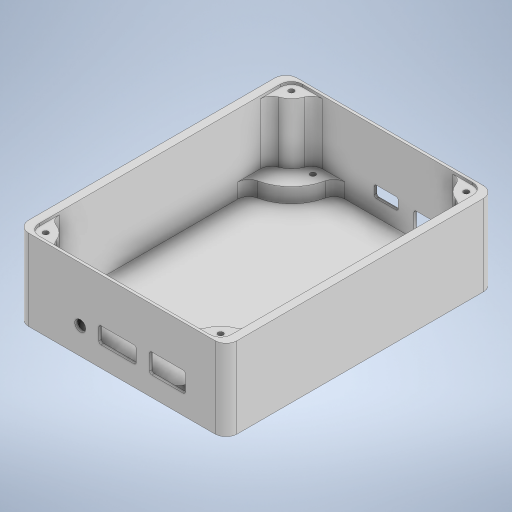
# Autodesk Inventor part: PrismGCNew
Saved by Autodesk Inventor 2024 (Build 280153000, 153)
## iProperties
Created: 2023-08-08
Part Number: PrismGCNew
Material: 常规
Document SubType Name: Modeling
Designer: liyuxuan
Density: 1 g/cm^3
Appearance: 默认
Author: liyuxuan
Autodesk Inventor part; units mm, degrees
ref_plane "YZ Plane" through (0, 0, 0) normal (1, 0, 0) x (0, 1, 0)
ref_plane "XZ Plane" through (0, 0, 0) normal (0, 1, 0) x (-1, 0, 0)
ref_plane "XY Plane" through (0, 0, 0) normal (0, 0, 1) x (1, 0, 0)
sketch "草图1" plane through (0, 0, 0) normal (0, 1, 0) x (-1, 0, 0)
  line L0 (-47.7, 61.39) -> (47.7, 61.39)
  line L1 (47.7, 61.39) -> (47.7, -61.39)
  line L2 (47.7, -61.39) -> (-47.7, -61.39)
  line L3 (-47.7, -61.39) -> (-47.7, 61.39)
  line L4 (-47.7, 61.39) -> (47.7, -61.39) construction
  line L5 (47.7, 61.39) -> (-47.7, -61.39) construction
  line L6 (-44, 60.19) -> (44, 60.19)
  line L7 (44, 60.19) -> (44, -60.19)
  line L8 (44, -60.19) -> (-44, -60.19)
  line L9 (-44, -60.19) -> (-44, 60.19)
  line L10 (-44, 60.19) -> (44, -60.19) construction
  line L11 (44, 60.19) -> (-44, -60.19) construction
  arc A0 (24, 60.19) -> (44, 40.19) centre (44, 60.19) ccw
  line L12 (44, 60.19) -> (24, 60.19) construction
  line L13 (44, 60.19) -> (44, 40.19) construction
  arc A1 (34, 60.19) -> (44, 50.19) centre (44, 60.19) ccw
  line L14 (44, 60.19) -> (34, 60.19) construction
  line L15 (44, 60.19) -> (44, 50.19) construction
  line L16 (44, 0) -> (-44, 0)
  line L17 (0, 60.19) -> (0, -60.19)
  circle A2 centre (40, 56.19) radius 1.25
  circle A3 centre (29.848, 55.88) radius 1.25
  arc A4 (44, -40.19) -> (24, -60.19) centre (44, -60.19) ccw
  arc A5 (44, -50.19) -> (34, -60.19) centre (44, -60.19) ccw
  circle A6 centre (40, -56.19) radius 1.25
  circle A7 centre (29.848, -55.88) radius 1.25
  arc A8 (-44, 40.19) -> (-24, 60.19) centre (-44, 60.19) ccw
  arc A9 (-44, 50.19) -> (-34, 60.19) centre (-44, 60.19) ccw
  circle A10 centre (-40, 56.19) radius 1.25
  circle A11 centre (-29.848, 55.88) radius 1.25
  arc A12 (-24, -60.19) -> (-44, -40.19) centre (-44, -60.19) ccw
  circle A13 centre (-29.848, -55.88) radius 1.25
  arc A14 (-34, -60.19) -> (-44, -50.19) centre (-44, -60.19) ccw
  circle A15 centre (-40, -56.19) radius 1.25
  point P0 (0, 0)
  point P1 (-44, -50.19)
  point P2 (-34, -60.19)
  point P3 (-24, -60.19)
  point P4 (-44, -40.19)
  point P5 (-34, 60.19)
  point P6 (-44, 50.19)
  point P7 (-44, 40.19)
  point P8 (-24, 60.19)
  point P9 (44, -50.19)
  dimension "d0" = 122.78
  dimension "d1" = 95.4
  dimension "d2" = 120.38
  dimension "d3" = 88
  dimension "d4" = 20
  dimension "d5" = 90
  dimension "d6" = 10
  dimension "d7" = 90
  dimension "d8" = 55.88
  dimension "d9" = 29.848
  dimension "d10" = 4
  dimension "d11" = 4
  dimension "d12" = 2.5
  dimension "d13" = 2.5
  constraints: 36 end point, 30 symmetric about line, 16 centre point, 16 point on circle, 13 coincident, 9 midpoint, 4 parallel, 2 horizontal, 2 perpendicular, 1 point on line, 12 other
  measures "d0" distance of L0.end L1.end
  measures "d1" distance of L0.start L0.end
  measures "d2" distance of L6.end L7.end
  measures "d3" distance of L6.start L6.end
  measures "d4" radius of A0
  measures "d5" angle of L12 L13
  measures "d6" radius of A1
  measures "d7" angle of L14 L15
  measures "d8" vertical distance of point (0, 0) point (29.848, 55.88)
  measures "d9" horizontal distance of point (29.848, 55.88) point (0, 0)
  measures "d10" distance from line of L12 point (40, 56.19)
  measures "d11" distance from line of L7 point (40, 56.19)
  measures "d12" diameter of A2
  measures "d13" diameter of A3
extrude "拉伸1" add sketch "草图1" along normal blind 37 contours L0 L1 L2 L3
extrude "拉伸2" add sketch "草图1" along normal blind 1.2 contours L6 A9 L9 | L6 A8 L9 A9 | L6 L17 L16 L9 A8 | L6 A0 L7 L16 L17 | L16 L17 L8 A12 L9 | L6 A1 L7 A0 | L16 L7 A4 L8 L17 | A12 L8 A14 L9 | L6 L7 A1 | A14 L8 L9 | L7 A5 L8 A4 | L7 L8 A5 | A2 | A3 | A6 | A7 | A10 | A11 | A13 | A15
extrude "拉伸3" add sketch "草图1" along normal blind 8 contours L6 A8 L9 A9 | L6 A1 L7 A0 | A12 L8 A14 L9 | L7 A5 L8 A4 | A3 | A7 | A11 | A13
extrude "拉伸4" add sketch "草图1" along normal blind 35.8 contours L6 A9 L9 | L6 L7 A1 | A14 L8 L9 | L7 L8 A5 | A2 | A6 | A10 | A15
sketch "草图3" plane through (0, 8, 0) normal (0, 1, 0) x (1, 0, 0)
  arc A0 (44, -50.19) -> (34, -60.19) centre (44, -60.19) ccw projected
  line L0 (44, -40.19) -> (44, -50.19) projected
  arc A1 (44, -40.19) -> (24, -60.19) centre (44, -60.19) ccw projected
  line L1 (-24, -60.19) -> (24, -60.19) projected
  arc A2 (-24, -60.19) -> (-44, -40.19) centre (-44, -60.19) ccw projected
  line L2 (-44, 40.19) -> (-44, -40.19) projected
  arc A3 (-44, 40.19) -> (-24, 60.19) centre (-44, 60.19) ccw projected
  line L3 (24, 60.19) -> (-24, 60.19) projected
  line L4 (34, 60.19) -> (24, 60.19) projected
  arc A4 (34, 60.19) -> (44, 50.19) centre (44, 60.19) ccw projected
  line L5 (44, 50.19) -> (44, 40.19) projected
  arc A5 (24, 60.19) -> (44, 40.19) centre (44, 60.19) ccw projected
  line L6 (24, -60.19) -> (34, -60.19) projected
  line L7 (44, -40.19) -> (44, 40.19) projected
  line L8 (-34, -60.19) -> (-24, -60.19) projected
  arc A6 (-34, -60.19) -> (-44, -50.19) centre (-44, -60.19) ccw projected
  line L9 (-44, -50.19) -> (-44, -40.19) projected
  line L10 (-44, 40.19) -> (-44, 50.19) projected
  arc A7 (-44, 50.19) -> (-34, 60.19) centre (-44, 60.19) ccw projected
  line L11 (-24, 60.19) -> (-34, 60.19) projected
  line L12 (47.7, 61.39) -> (47.7, -61.39) projected
  line L13 (47.7, -61.39) -> (-47.7, -61.39) projected
  line L14 (-47.7, -61.39) -> (-47.7, 61.39) projected
  line L15 (-47.7, 61.39) -> (47.7, 61.39) projected
  line L16 (-44, 0) -> (44, 0) projected
  line L17 (0, -60.19) -> (0, 60.19) projected
  arc A8 (-24, -60.19) -> (-44, -40.19) centre (-44, -60.19) ccw projected
  arc A9 (44, -50.19) -> (34, -60.19) centre (44, -60.19) ccw projected
  line L18 (44, -40.19) -> (44, -50.19) projected
  arc A10 (44, -40.19) -> (24, -60.19) centre (44, -60.19) ccw projected
  line L19 (-24, -60.19) -> (24, -60.19) projected
  arc A11 (-24, -60.19) -> (-44, -40.19) centre (-44, -60.19) ccw projected
  line L20 (-44, 40.19) -> (-44, -40.19) projected
  arc A12 (-44, 40.19) -> (-24, 60.19) centre (-44, 60.19) ccw projected
  line L21 (24, 60.19) -> (-24, 60.19) projected
  line L22 (34, 60.19) -> (24, 60.19) projected
  arc A13 (34, 60.19) -> (44, 50.19) centre (44, 60.19) ccw projected
  line L23 (44, 50.19) -> (44, 40.19) projected
  arc A14 (24, 60.19) -> (44, 40.19) centre (44, 60.19) ccw projected
  line L24 (24, -60.19) -> (34, -60.19) projected
  line L25 (44, -40.19) -> (44, 40.19) projected
  line L26 (-34, -60.19) -> (-24, -60.19) projected
  arc A15 (-34, -60.19) -> (-44, -50.19) centre (-44, -60.19) ccw projected
  line L27 (-44, -50.19) -> (-44, -40.19) projected
  line L28 (-44, 40.19) -> (-44, 50.19) projected
  arc A16 (-44, 50.19) -> (-34, 60.19) centre (-44, 60.19) ccw projected
  line L29 (-24, 60.19) -> (-34, 60.19) projected
  line L30 (47.7, 61.39) -> (47.7, -61.39) projected
  line L31 (47.7, -61.39) -> (-47.7, -61.39) projected
  line L32 (-47.7, -61.39) -> (-47.7, 61.39) projected
  line L33 (-47.7, 61.39) -> (47.7, 61.39) projected
  point P0 (0, 0)
  point P1 (-29.848, -55.88)
  point P2 (-29.848, -55.88)
  point P3 (-29.848, 55.88)
  point P4 (29.848, -55.88)
  point P5 (29.848, 55.88)
  constraints: 3 symmetric about line, 1 coincident
hole "孔3" at (-29.848, 8, 55.88) at (-29.848, 8, -55.88) at (29.848, 8, 55.88) at (29.848, 8, -55.88) direction (0, -1, 0) diameter 2.459 depth 6 tip angle 118 thread size "M3x0.5" designation "M3" class "6H" standard "GB Metric profile"
sketch "草图6" plane through (0, 35.8, 0) normal (0, 1, 0) x (1, 0, 0)
  arc A0 (44, -40.19) -> (24, -60.19) centre (44, -60.19) ccw projected
  line L0 (44, 40.19) -> (44, -40.19) projected
  arc A1 (24, 60.19) -> (44, 40.19) centre (44, 60.19) ccw projected
  line L1 (-24, 60.19) -> (24, 60.19) projected
  arc A2 (-44, 40.19) -> (-24, 60.19) centre (-44, 60.19) ccw projected
  line L2 (-44, -40.19) -> (-44, 40.19) projected
  arc A3 (-24, -60.19) -> (-44, -40.19) centre (-44, -60.19) ccw projected
  line L3 (24, -60.19) -> (-24, -60.19) projected
  arc A4 (44, -50.19) -> (34, -60.19) centre (44, -60.19) ccw projected
  line L4 (44, -50.19) -> (44, -60.19) projected
  line L5 (44, -60.19) -> (34, -60.19) projected
  line L6 (-34, -60.19) -> (34, -60.19) projected
  arc A5 (-34, -60.19) -> (-44, -50.19) centre (-44, -60.19) ccw projected
  line L7 (-44, 50.19) -> (-44, -50.19) projected
  arc A6 (-44, 50.19) -> (-34, 60.19) centre (-44, 60.19) ccw projected
  line L8 (34, 60.19) -> (-34, 60.19) projected
  arc A7 (34, 60.19) -> (44, 50.19) centre (44, 60.19) ccw projected
  line L9 (44, -50.19) -> (44, 50.19) projected
  line L10 (-34, -60.19) -> (-44, -60.19) projected
  line L11 (-44, -60.19) -> (-44, -50.19) projected
  line L12 (-44, 50.19) -> (-44, 60.19) projected
  line L13 (-44, 60.19) -> (-34, 60.19) projected
  line L14 (34, 60.19) -> (44, 60.19) projected
  line L15 (44, 60.19) -> (44, 50.19) projected
  line L16 (47.7, 61.39) -> (47.7, -61.39) projected
  line L17 (47.7, -61.39) -> (-47.7, -61.39) projected
  line L18 (-47.7, -61.39) -> (-47.7, 61.39) projected
  line L19 (-47.7, 61.39) -> (47.7, 61.39) projected
  arc A8 (44, -50.19) -> (34, -60.19) centre (44, -60.19) ccw projected
  line L20 (44, -50.19) -> (44, -60.19) projected
  line L21 (44, -60.19) -> (34, -60.19) projected
  line L22 (-34, -60.19) -> (34, -60.19) projected
  arc A9 (-34, -60.19) -> (-44, -50.19) centre (-44, -60.19) ccw projected
  line L23 (-44, 50.19) -> (-44, -50.19) projected
  arc A10 (-44, 50.19) -> (-34, 60.19) centre (-44, 60.19) ccw projected
  line L24 (34, 60.19) -> (-34, 60.19) projected
  arc A11 (34, 60.19) -> (44, 50.19) centre (44, 60.19) ccw projected
  line L25 (44, -50.19) -> (44, 50.19) projected
  line L26 (-34, -60.19) -> (-44, -60.19) projected
  line L27 (-44, -60.19) -> (-44, -50.19) projected
  line L28 (-44, 50.19) -> (-44, 60.19) projected
  line L29 (-44, 60.19) -> (-34, 60.19) projected
  line L30 (34, 60.19) -> (44, 60.19) projected
  line L31 (44, 60.19) -> (44, 50.19) projected
  line L32 (-44, 0) -> (44, 0) projected
  line L33 (0, -60.19) -> (0, 60.19) projected
  line L34 (47.7, 61.39) -> (47.7, -61.39) projected
  line L35 (47.7, -61.39) -> (-47.7, -61.39) projected
  line L36 (-47.7, -61.39) -> (-47.7, 61.39) projected
  line L37 (-47.7, 61.39) -> (47.7, 61.39) projected
  point P0 (0, 0)
  point P1 (-40, -56.19)
  point P2 (-40, 56.19)
  point P3 (40, -56.19)
  point P4 (40, 56.19)
  dimension "d50" = 4
  dimension "d51" = 4
  constraints: 3 symmetric about line
  measures "d50" distance from line of L10 point (-40, -56.19)
  measures "d51" distance from line of L11 point (-40, -56.19)
hole "孔5" at (-40, 35.8, 56.19) at (-40, 35.8, -56.19) at (40, 35.8, 56.19) at (40, 35.8, -56.19) direction (0, -1, 0) diameter 2.459 depth 6 tip angle 118 thread size "M3x0.5" designation "M3" class "6H" standard "GB Metric profile"
fillet "面圆角1" radius 5 1 edges at (44, 36.4, 60.19)
fillet "面圆角2" radius 5 1 edges at (47.7, 18.5, 61.39)
fillet "面圆角3" radius 5 1 edges at (-44, 36.4, -60.19)
fillet "面圆角4" radius 5 1 edges at (44, 36.4, -60.19)
fillet "面圆角5" radius 5 1 edges at (-44, 36.4, 60.19)
fillet "面圆角6" radius 5 1 edges at (47.7, 18.5, -61.39)
fillet "面圆角7" radius 5 1 edges at (-47.7, 18.5, 61.39)
fillet "面圆角8" radius 5 1 edges at (-47.7, 18.5, -61.39)
fillet "面圆角9" radius 5 1 edges at (-44, 21.9, -50.19)
fillet "面圆角10" radius 5 1 edges at (-34, 21.9, -60.19)
fillet "面圆角11" radius 5 1 edges at (-44, 4.6, -40.19)
fillet "面圆角12" radius 5 1 edges at (-24, 4.6, -60.19)
fillet "面圆角13" radius 5 1 edges at (24, 4.6, -60.19)
fillet "面圆角14" radius 5 1 edges at (44, 4.6, -40.19)
fillet "面圆角15" radius 5 1 edges at (34, 21.9, -60.19)
fillet "面圆角16" radius 5 1 edges at (44, 21.9, -50.19)
fillet "面圆角17" radius 5 1 edges at (44, 21.9, 50.19)
fillet "面圆角18" radius 5 1 edges at (34, 21.9, 60.19)
fillet "面圆角19" radius 5 1 edges at (44, 4.6, 40.19)
fillet "面圆角20" radius 5 1 edges at (24, 4.6, 60.19)
fillet "面圆角21" radius 5 1 edges at (-24, 4.6, 60.19)
fillet "面圆角22" radius 5 1 edges at (-44, 4.6, 40.19)
fillet "面圆角23" radius 5 1 edges at (-34, 21.9, 60.19)
fillet "面圆角24" radius 5 1 edges at (-44, 21.9, 50.19)
sketch "草图7" plane through (42.7, 0, 61.39) normal (0, 0, 1) x (1, 0, 0)
  line L0 (-83.3667, 8) -> (-83.3667, 8) projected
  line L1 (-83.3667, 8) -> (-77.2719, 8) projected
  line L2 (-77.2719, 8) -> (-72.5579, 8) projected
  line L3 (-62.2051, 8) -> (-72.5579, 8) projected
  line L4 (-62.2051, 8) -> (-67.1041, 8) projected
  line L5 (-67.1041, 8) -> (-86.7, 8) projected
  line L6 (-86.7, 8) -> (-86.7, 8) projected
  line L7 (-73.7775, 8) -> (-71.3185, 8) projected
  line L8 (-12.8421, 8) -> (-8.1281, 8) projected
  line L9 (-8.1281, 8) -> (-2.0333, 8) projected
  line L10 (-2.0333, 8) -> (1.3, 8) projected
  line L11 (1.3, 8) -> (-2.7, 8) projected
  line L12 (-2.7, 8) -> (-18.2959, 8) projected
  line L13 (-23.1949, 8) -> (-18.2959, 8) projected
  line L14 (-12.8421, 8) -> (-23.1949, 8) projected
  line L15 (-14.0815, 8) -> (-11.6225, 8) projected
  line L16 (-14.0815, 8) -> (-11.6225, 8) projected
  line L17 (-73.7775, 8) -> (-71.3185, 8) projected
  line L18 (-86.7, 1.2) -> (-82.7, 1.2) projected
  line L19 (-82.7, 1.2) -> (-67.1041, 1.2) projected
  line L20 (-67.1041, 1.2) -> (-62.2051, 1.2) projected
  line L21 (-23.1949, 1.2) -> (-62.2051, 1.2) projected
  line L22 (-23.1949, 1.2) -> (-18.2959, 1.2) projected
  line L23 (-18.2959, 1.2) -> (-2.7, 1.2) projected
  line L24 (-2.7, 1.2) -> (1.3, 1.2) projected
  line L25 (1.3, 1.2) -> (-2.7, 1.2) projected
  line L26 (-2.7, 1.2) -> (-18.2959, 1.2) projected
  line L27 (-18.2959, 1.2) -> (-23.1949, 1.2) projected
  line L28 (-62.2051, 1.2) -> (-23.1949, 1.2) projected
  line L29 (-62.2051, 1.2) -> (-67.1041, 1.2) projected
  line L30 (-67.1041, 1.2) -> (-82.7, 1.2) projected
  line L31 (-82.7, 1.2) -> (-86.7, 1.2) projected
  line L32 (-90.4, 37) -> (-85.4, 37) projected
  line L33 (0, 37) -> (0, 0) projected
  line L34 (-85.4, 37) -> (0, 0)
  line L35 (-85.4, 0) -> (-85.4, 37) projected
  line L36 (0, 37) -> (-84.5262, -1.8989)
  line L37 (-85.4, 9.6) -> (0, 9.6)
  line L38 (-40.2, 18.5) -> (-42.7, 9.6)
  line L39 (-86.7, 8) -> (-83.3667, 8) projected
  line L40 (-86.7, 8) -> (-2.7, 8)
  line L41 (-13.585, 18.05) -> (-29.985, 18.05)
  line L42 (-29.985, 18.05) -> (-29.985, 8.95)
  line L43 (-29.985, 8.95) -> (-13.585, 8.95)
  line L44 (-13.585, 8.95) -> (-13.585, 18.05)
  line L45 (-13.585, 18.05) -> (-29.985, 8.95) construction
  line L46 (-29.985, 18.05) -> (-13.585, 8.95) construction
  line L47 (-44.645, 16.85) -> (-44.645, 9.3)
  line L48 (-36.095, 16.85) -> (-53.195, 16.85)
  line L49 (-53.195, 16.85) -> (-53.195, 9.3)
  line L50 (-53.195, 9.3) -> (-36.095, 9.3)
  line L51 (-36.095, 9.3) -> (-36.095, 16.85)
  line L52 (-36.095, 16.85) -> (-53.195, 9.3) construction
  line L53 (-53.195, 16.85) -> (-36.095, 9.3) construction
  circle A0 centre (-61.663, 12.1) radius 2.5
  point P0 (-42.7, 0)
  point P1 (-24.285, 9.6)
  point P2 (-21.785, 8)
  point P3 (-21.785, 8.95)
  point P4 (-21.785, 18.05)
  point P5 (-21.785, 13.5)
  point P6 (-47.145, 9.6)
  point P7 (-44.645, 8)
  point P8 (-44.645, 13.075)
  point P9 (-64.163, 9.6)
  point P10 (-61.663, 8)
  dimension "d84" = 1.6
  dimension "d85" = 18.415
  dimension "d86" = 0.95
  dimension "d87" = 10.05
  dimension "d88" = 16.4
  dimension "d89" = 4.445
  dimension "d90" = 1.3
  dimension "d91" = 8.85
  dimension "d92" = 17.1
  dimension "d93" = 21.463
  dimension "d94" = 4.1
  dimension "d95" = 5
  constraints: 34 end point, 8 point on line, 6 midpoint, 4 parallel, 3 perpendicular, 2 coincident, 2 horizontal, 1 centre point, 1 collinear, 1 vertical, 5 other
  measures "d84" distance between parallel lines of L37 L3
  measures "d85" distance of point (-24.285, 9.6) L38.end
  measures "d86" distance of point (-21.785, 8.95) point (-21.785, 8)
  measures "d87" distance of point (-21.785, 8) point (-21.785, 18.05)
  measures "d88" distance of L43.end L42.end
  measures "d89" distance of point (-47.145, 9.6) point (-42.7, 9.6)
  measures "d90" distance of L47.end point (-44.645, 8)
  measures "d91" distance of point (-44.645, 8) L47.start
  measures "d92" distance of L50.end L49.end
  measures "d93" distance of point (-64.163, 9.6) L38.end
  measures "d94" distance of point (-61.663, 8) point (-61.663, 12.1)
  measures "d95" diameter of A0
extrude "拉伸5" cut sketch "草图7" against normal blind 20 contours A0 | L48 L38 L37 L47 L36 | L36 L47 L48 | L49 L48 L47 L36 | L36 L47 L37 L49 | L37 L47 L50 L49 | L48 L51 L34 | L34 L51 L37 L38 L48 | L37 L51 L50 L47 | L42 L41 L44 L37 L34 | L34 L37 L42 | L44 L43 L34 L37 | L43 L42 L37 L34
fillet "面圆角25" radius 1 1 edges at (-10.495, 16.85, 60.79)
fillet "面圆角26" radius 1 1 edges at (6.605, 16.85, 60.79)
fillet "面圆角27" radius 1 1 edges at (6.605, 9.3, 60.79)
fillet "面圆角28" radius 1 1 edges at (-10.495, 9.3, 60.79)
fillet "面圆角29" radius 1 1 edges at (12.715, 18.05, 60.79)
fillet "面圆角30" radius 1 1 edges at (29.115, 18.05, 60.79)
fillet "面圆角31" radius 1 1 edges at (29.115, 8.95, 60.79)
fillet "面圆角32" radius 1 1 edges at (12.715, 8.95, 60.79)
sketch "草图8" plane through (42.7, 0, -61.39) normal (0, 0, -1) x (-1, 0, 0)
  point P0 (42.7, 0)
sketch "草图9" plane through (42.7, 0, -61.39) normal (0, 0, -1) x (-1, 0, 0)
  line L0 (18.2959, 8) -> (2.7, 8) projected
  line L1 (-1.3, 8) -> (2.0333, 8) projected
  line L2 (2.0333, 8) -> (8.1281, 8) projected
  line L3 (8.1281, 8) -> (12.8421, 8) projected
  line L4 (23.1949, 8) -> (12.8421, 8) projected
  line L5 (23.1949, 8) -> (18.2959, 8) projected
  line L6 (18.2959, 8) -> (2.7, 8) projected
  line L7 (-1.3, 8) -> (2.7, 8) projected
  line L8 (11.6225, 8) -> (14.0815, 8) projected
  line L9 (72.5579, 8) -> (77.2719, 8) projected
  line L10 (77.2719, 8) -> (83.3667, 8) projected
  line L11 (83.3667, 8) -> (86.7, 8) projected
  line L12 (86.7, 8) -> (82.7, 8) projected
  line L13 (82.7, 8) -> (67.1041, 8) projected
  line L14 (62.2051, 8) -> (67.1041, 8) projected
  line L15 (72.5579, 8) -> (62.2051, 8) projected
  line L16 (71.3185, 8) -> (73.7775, 8) projected
  line L17 (82.7, 8) -> (67.1041, 8) projected
  line L18 (86.7, 1.2) -> (82.7, 1.2) projected
  line L19 (82.7, 1.2) -> (67.1041, 1.2) projected
  line L20 (67.1041, 1.2) -> (62.2051, 1.2) projected
  line L21 (23.1949, 1.2) -> (62.2051, 1.2) projected
  line L22 (23.1949, 1.2) -> (18.2959, 1.2) projected
  line L23 (18.2959, 1.2) -> (2.7, 1.2) projected
  line L24 (2.7, 1.2) -> (-1.3, 1.2) projected
  line L25 (-1.3, 1.2) -> (2.7, 1.2) projected
  line L26 (2.7, 1.2) -> (18.2959, 1.2) projected
  line L27 (18.2959, 1.2) -> (23.1949, 1.2) projected
  line L28 (62.2051, 1.2) -> (23.1949, 1.2) projected
  line L29 (62.2051, 1.2) -> (67.1041, 1.2) projected
  line L30 (67.1041, 1.2) -> (82.7, 1.2) projected
  line L31 (82.7, 1.2) -> (86.7, 1.2) projected
  line L32 (0, 0) -> (0, 37) projected
  line L33 (85.4, 37) -> (85.4, 0) projected
  line L34 (0, 37) -> (85.4, 37) projected
  line L35 (0, 1.2) -> (85.4, 1.2)
  line L36 (0, 8) -> (85.4, 8)
  line L37 (0, 9.6) -> (85.4, 9.6)
  line L38 (0, 8.8) -> (85.4, 8.8)
  line L39 (42.7, 19.1) -> (42.7, 8)
  line L40 (16.398, 3.54) -> (30.648, 3.54)
  line L41 (30.648, 3.54) -> (30.648, 12.74)
  line L42 (30.648, 12.74) -> (16.398, 12.74)
  line L43 (16.398, 12.74) -> (16.398, 3.54)
  line L44 (48.835, 13.9) -> (37.835, 13.9)
  line L45 (37.835, 13.9) -> (37.835, 8.6)
  line L46 (37.835, 8.6) -> (48.835, 8.6)
  line L47 (48.835, 8.6) -> (48.835, 13.9)
  line L48 (48.835, 13.9) -> (37.835, 8.6) construction
  line L49 (37.835, 13.9) -> (48.835, 8.6) construction
  line L50 (16.398, 12.74) -> (30.648, 12.74)
  line L51 (30.648, 12.74) -> (30.648, 3.54)
  line L52 (30.648, 3.54) -> (16.398, 3.54)
  line L53 (16.398, 3.54) -> (16.398, 12.74)
  point P0 (42.7, 0)
  point P1 (84.7, 8)
  point P2 (23.523, 8.8)
  point P3 (42.7, 8.8)
  point P4 (23.523, 12.74)
  point P5 (23.523, 3.54)
  point P6 (43.335, 8)
  point P7 (43.335, 9.6)
  point P8 (43.335, 11.25)
  point P9 (16.398, 3.54)
  dimension "d106" = 1.6
  dimension "d107" = 0.8
  dimension "d108" = 19.177
  dimension "d109" = 3.94
  dimension "d110" = 5.26
  dimension "d111" = 7.125
  dimension "d112" = 7.125
  dimension "d113" = 0.635
  dimension "d114" = 1.65
  dimension "d115" = 11
  dimension "d116" = 5.3
  constraints: 38 end point, 15 point on line, 6 parallel, 6 perpendicular, 5 midpoint, 4 horizontal, 2 coincident, 1 collinear
  measures "d106" distance from line of L39.end L37
  measures "d107" distance from line of point (84.7, 8) L38
  measures "d108" distance of point (42.7, 8.8) point (23.523, 8.8)
  measures "d109" distance of point (23.523, 12.74) point (23.523, 8.8)
  measures "d110" distance of point (23.523, 3.54) point (23.523, 8.8)
  measures "d111" distance of L41.end point (23.523, 12.74)
  measures "d112" distance of point (23.523, 3.54) L40.start
  measures "d113" distance of L39.end point (43.335, 8)
  measures "d114" distance of point (43.335, 9.6) point (43.335, 11.25)
  measures "d115" distance of L46.end L45.end
  measures "d116" distance of L45.end L44.end
extrude "拉伸6" cut sketch "草图9" against normal blind 20 contours L43 L38 L41 L36 L4 L0 | L0 L4 L36 L41 L40 L43 | L43 L37 L41 L38 | L43 L42 L41 L37 | L45 L37 L39 L38 | L38 L39 L46 L45 | L39 L37 L47 L38 | L38 L47 L46 L39 | L45 L44 L39 L37 | L39 L44 L47 L37
fillet "面圆角33" radius 1 1 edges at (12.052, 3.54, -60.79)
fillet "面圆角34" radius 1 1 edges at (26.302, 3.54, -56.1322)
fillet "面圆角35" radius 1 1 edges at (26.302, 12.74, -60.79)
fillet "面圆角36" radius 1 1 edges at (12.052, 12.74, -60.79)
fillet "面圆角37" radius 1 1 edges at (4.865, 13.9, -60.79)
fillet "面圆角38" radius 1 1 edges at (-6.135, 13.9, -60.79)
fillet "面圆角39" radius 1 1 edges at (-6.135, 8.6, -60.79)
fillet "面圆角40" radius 1 1 edges at (4.865, 8.6, -60.79)
